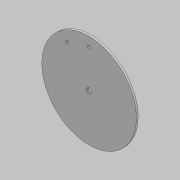
# Autodesk Inventor part: RotatoryDisk
Saved by Autodesk Inventor 2018 (Build 220112000, 112)
## iProperties
Created: 2019-06-28
Part Number: RotatoryDisk
Material: Generic
Document SubType Name: Modeling
Designer: mkivekas
Density: 1 g/cm^3
Appearance: Default
Author: mkivekas
Autodesk Inventor part; units mm, degrees
ref_plane "YZ Plane" through (0, 0, 0) normal (1, 0, 0) x (0, 1, 0)
ref_plane "XZ Plane" through (0, 0, 0) normal (0, 1, 0) x (-1, 0, 0)
ref_plane "XY Plane" through (0, 0, 0) normal (0, 0, 1) x (1, 0, 0)
sketch "Sketch1" plane through (0, 0, 0) normal (0, 1, 0) x (-1, 0, 0)
  circle A0 centre (0, 0) radius 50
  circle A1 centre (0, 0) radius 40
  point P0 (0, 40)
  point P1 (22.9431, 32.7661)
  dimension "d0" = 100
  dimension "d3" = 10
  dimension "d4" = 35
  constraints: 3 coincident, 2 centre point, 2 point on circle
  measures "d0" diameter of A0
  measures "d3" radial gap between concentric circles of A0 A1
extrude "Extrusion1" add sketch "Sketch1" along normal blind 2 contours A0 | A1
hole "Hole1" at (0, 0, 40) at (-22.9431, 0, 32.7661) direction (0, 1, 0) diameter 3 depth 8 tip angle 118
hole "Hole2" at (0, 0, 0) direction (0, 1, 0) diameter 5 depth 8 tip angle 118
body "Solid1"
